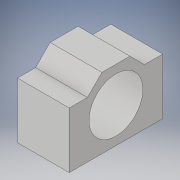
# Autodesk Inventor part: spindleMount
Saved by Autodesk Inventor 2019 (Build 230136000, 136)
## iProperties
Created: 2019-05-08
Part Number: spindleMount
Material: Generic
Document SubType Name: Modeling
Designer: Alex Jones
Density: 1 g/cm^3
Appearance: Default
Author: Alex Jones
Autodesk Inventor part; units mm, degrees
ref_plane "YZ Plane" through (0, 0, 0) normal (1, 0, 0) x (0, 1, 0)
ref_plane "XZ Plane" through (0, 0, 0) normal (0, 1, 0) x (-1, 0, 0)
ref_plane "XY Plane" through (0, 0, 0) normal (0, 0, 1) x (1, 0, 0)
sketch "Sketch1" plane through (0, 0, 0) normal (1, 0, 0) x (0, 1, 0)
  line L0 (0, 0) -> (257.364, 0) construction
  line L1 (0, 0) -> (0, 45)
  line L2 (0, 45) -> (54, 45)
  line L3 (54, 0) -> (54, 27.5) construction
  line L4 (54, 45) -> (54, 27.5)
  line L5 (68, 0) -> (68, 13.5)
  line L6 (54, 27.5) -> (68, 13.5)
  circle A0 centre (34, 0) radius 26
  line L7 (0, 0) -> (0, -45)
  line L8 (0, -45) -> (54, -45)
  line L9 (54, -45) -> (54, -27.5)
  line L10 (68, 0) -> (68, -13.5)
  line L11 (54, -27.5) -> (68, -13.5)
  dimension "d0" = 45
  dimension "d1" = 54
  dimension "d2" = 27.5
  dimension "d4" = 13.5
  dimension "d5" = 68
  dimension "d6" = 52
  dimension "d7" = 34
  constraints: 24 end point, 4 symmetric about line, 3 point on line, 2 horizontal, 2 vertical, 1 centre point, 1 perpendicular
  measures "d0" distance of L0.start L1.end
  measures "d1" distance of L1.end L2.end
  measures "d2" distance of L3.start L3.end
  measures "d4" distance of L5.start L5.end
  measures "d5" distance between parallel lines of L1 L5
  measures "d6" diameter of A0
  measures "d7" distance from line of L1 A0.centre
extrude "Extrusion1" add sketch "Sketch1" along normal blind 50
body "Solid1"
